Autodesk Fusion 360 part; units mm, degrees
note: some values were not read from the file. Set by a fixed rule: which sketch regions a step uses.
(part 27 of 59)
  spline S36 degree 5 poles (-3.9508, -16.2753) (-3.9508, -16.2754) (-3.9508, -16.2756) (-3.9509, -16.2759) (-3.9509, -16.2764) (-3.951, -16.2772) (-3.9511, -16.278) (-3.9512, -16.279) (-3.9514, -16.2801) (-3.9515, -16.2813) (-3.9517, -16.2826) (-3.9518, -16.284) (-3.952, -16.2855) (-3.9522, -16.2871) (-3.9523, -16.2889) (-3.9525, -16.2907) (-3.9527, -16.2926) (-3.9529, -16.2946) (-3.9531, -16.2968) (-3.9534, -16.299) (-3.9536, -16.3013) (-3.9538, -16.3037) (-3.954, -16.3063) (-3.9543, -16.3089) (-3.9545, -16.3116) (-3.9547, -16.3144) (-3.955, -16.3172) (-3.9552, -16.3202) (-3.9555, -16.3233) (-3.9557, -16.3264) (-3.9559, -16.3297) (-3.9562, -16.333) (-3.9564, -16.3364) (-3.9567, -16.3399) (-3.9569, -16.3435) (-3.9572, -16.3472) (-3.9574, -16.3509) (-3.9577, -16.3547) (-3.9579, -16.3586) (-3.9581, -16.3626) (-3.9584, -16.3667) (-3.9586, -16.3709) (-3.9588, -16.3751) (-3.959, -16.3794) (-3.9593, -16.3838) (-3.9595, -16.3882) (-3.9597, -16.3928) (-3.9599, -16.3974) (-3.9601, -16.4021) (-3.9603, -16.4068) (-3.9605, -16.4117) (-3.9607, -16.4166) (-3.9609, -16.4215) (-3.961, -16.4266) (-3.9612, -16.4317) (-3.9614, -16.4369) (-3.9615, -16.4422) (-3.9617, -16.4475) (-3.9618, -16.4529) (-3.962, -16.4584) (-3.9621, -16.4639) (-3.9622, -16.4695) (-3.9623, -16.4752) (-3.9624, -16.4809) (-3.9625, -16.4867) (-3.9626, -16.4926) (-3.9627, -16.4985) (-3.9627, -16.5045) (-3.9628, -16.5106) (-3.9629, -16.5167) (-3.9629, -16.5229) (-3.9629, -16.5291) (-3.9629, -16.5355) (-3.963, -16.5418) (-3.963, -16.5483) (-3.9629, -16.5548) (-3.9629, -16.5613) (-3.9629, -16.568) (-3.9628, -16.5746) (-3.9628, -16.5814) (-3.9627, -16.5882) (-3.9626, -16.595) (-3.9626, -16.6019) (-3.9625, -16.6089) (-3.9623, -16.6159) (-3.9622, -16.623) (-3.9621, -16.6302) (-3.9619, -16.6374) (-3.9618, -16.6446) (-3.9616, -16.6519) (-3.9614, -16.6593) (-3.9612, -16.6667) (-3.961, -16.6742) (-3.9607, -16.6817) (-3.9605, -16.6893) (-3.9603, -16.697) (-3.96, -16.7047) (-3.9597, -16.7124) (-3.9594, -16.7202) (-3.9591, -16.7281) (-3.9588, -16.736) (-3.9584, -16.7439) (-3.9581, -16.7519) (-3.9577, -16.76) (-3.9573, -16.7681) (-3.9569, -16.7763) (-3.9565, -16.7845) (-3.9561, -16.7927) (-3.9556, -16.801) (-3.9552, -16.8094) (-3.9547, -16.8178) (-3.9542, -16.8263) (-3.9537, -16.8348) (-3.9532, -16.8433) (-3.9526, -16.8519) (-3.9521, -16.8606) (-3.9515, -16.8693) (-3.9509, -16.878) (-3.9503, -16.8868) (-3.9497, -16.8957) (-3.9491, -16.9045) (-3.9484, -16.9135) (-3.9478, -16.9225) (-3.9471, -16.9315) (-3.9464, -16.9406) (-3.9457, -16.9497) (-3.9449, -16.9588) (-3.9442, -16.968) (-3.9434, -16.9773) (-3.9426, -16.9866) (-3.9418, -16.9959) (-3.941, -17.0053) (-3.9402, -17.0147) (-3.9393, -17.0242) (-3.9384, -17.0337) (-3.9375, -17.0433) (-3.9366, -17.0529) (-3.9357, -17.0625) (-3.9348, -17.0722) (-3.9338, -17.0819) (-3.9328, -17.0917) (-3.9318, -17.1015) (-3.9308, -17.1113) (-3.9297, -17.1212) (-3.9287, -17.1312) (-3.9276, -17.1411) (-3.9265, -17.1512) (-3.9254, -17.1612) (-3.9243, -17.1713) (-3.9231, -17.1814) (-3.922, -17.1916) (-3.9208, -17.2018) (-3.9196, -17.2121) (-3.9183, -17.2224) (-3.9171, -17.2327) (-3.9158, -17.2431) (-3.9145, -17.2535) (-3.9132, -17.264) (-3.9119, -17.2744) (-3.9106, -17.285) (-3.9092, -17.2955) (-3.9078, -17.3061) (-3.9064, -17.3168) (-3.905, -17.3274) (-3.9035, -17.3382) (-3.9021, -17.3489) (-3.9006, -17.3597) (-3.8991, -17.3705) (-3.8976, -17.3814) (-3.896, -17.3923) (-3.8945, -17.4032) (-3.8929, -17.4142) (-3.8913, -17.4252) (-3.8896, -17.4362) (-3.888, -17.4473) (-3.8863, -17.4584) (-3.8846, -17.4696) (-3.8829, -17.4807) (-3.8812, -17.492) (-3.8795, -17.5032) (-3.8777, -17.5145) (-3.8759, -17.5258) (-3.8741, -17.5372) (-3.8722, -17.5486) (-3.8704, -17.56) (-3.8685, -17.5714) (-3.8666, -17.5829) (-3.8647, -17.5944) (-3.8628, -17.606) (-3.8608, -17.6176) (-3.8588, -17.6292) (-3.8568, -17.6409) (-3.8548, -17.6525) (-3.8527, -17.6643) (-3.8507, -17.676) (-3.8486, -17.6878) (-3.8464, -17.6996) (-3.8443, -17.7115) (-3.8422, -17.7233) (-3.84, -17.7353) (-3.8378, -17.7472) (-3.8356, -17.7592) (-3.8333, -17.7712) (-3.831, -17.7832) (-3.8288, -17.7953) (-3.8264, -17.8074) (-3.8241, -17.8195) (-3.8217, -17.8317) (-3.8194, -17.8439) (-3.817, -17.8561) (-3.8145, -17.8683) (-3.8121, -17.8806) (-3.8096, -17.8929) (-3.8071, -17.9053) (-3.8046, -17.9176) (-3.8021, -17.93) (-3.7995, -17.9424) (-3.797, -17.9549) (-3.7943, -17.9674) (-3.7917, -17.9799) (-3.7891, -17.9924) (-3.7864, -18.005) (-3.7837, -18.0176) (-3.781, -18.0302) (-3.7782, -18.0429) (-3.7755, -18.0556) (-3.7727, -18.0683) (-3.7699, -18.081) (-3.767, -18.0938) (-3.7642, -18.1066) (-3.7613, -18.1194) (-3.7584, -18.1323) (-3.7555, -18.1451) (-3.7525, -18.158) (-3.7496, -18.171) (-3.7466, -18.1839) (-3.7435, -18.1969) (-3.7405, -18.2099) (-3.7374, -18.223) (-3.7343, -18.236) (-3.7312, -18.2491) (-3.7287, -18.2596) (-3.7268, -18.2675) (-3.7256, -18.2728) (-3.7249, -18.2754) knots 0 0 0 0 0 0 0.00416667 0.00833333 0.0125 0.01666667 0.02083333 0.025 0.02916667 0.03333333 0.0375 0.04166667 0.04583333 0.05 0.05416667 0.05833333 0.0625 0.06666667 0.07083333 0.075 0.07916667 0.08333333 0.0875 0.09166667 0.09583333 0.1 0.10416667 0.10833333 0.1125 0.11666667 0.12083333 0.125 0.12916667 0.13333333 0.1375 0.14166667 0.14583333 0.15 0.15416667 0.15833333 0.1625 0.16666667 0.17083333 0.175 0.17916667 0.18333333 0.1875 0.19166667 0.19583333 0.2 0.20416667 0.20833333 0.2125 0.21666667 0.22083333 0.225 0.22916667 0.23333333 0.2375 0.24166667 0.24583333 0.25 0.25416667 0.25833333 0.2625 0.26666667 0.27083333 0.275 0.27916667 0.28333333 0.2875 0.29166667 0.29583333 0.3 0.30416667 0.30833333 0.3125 0.31666667 0.32083333 0.325 0.32916667 0.33333333 0.3375 0.34166667 0.34583333 0.35 0.35416667 0.35833333 0.3625 0.36666667 0.37083333 0.375 0.37916667 0.38333333 0.3875 0.39166667 0.39583333 0.4 0.40416667 0.40833333 0.4125 0.41666667 0.42083333 0.425 0.42916667 0.43333333 0.4375 0.44166667 0.44583333 0.45 0.45416667 0.45833333 0.4625 0.46666667 0.47083333 0.475 0.47916667 0.48333333 0.4875 0.49166667 0.49583333 0.5 0.50416667 0.50833333 0.5125 0.51666667 0.52083333 0.525 0.52916667 0.53333333 0.5375 0.54166667 0.54583333 0.55 0.55416667 0.55833333 0.5625 0.56666667 0.57083333 0.575 0.57916667 0.58333333 0.5875 0.59166667 0.59583333 0.6 0.60416667 0.60833333 0.6125 0.61666667 0.62083333 0.625 0.62916667 0.63333333 0.6375 0.64166667 0.64583333 0.65 0.65416667 0.65833333 0.6625 0.66666667 0.67083333 0.675 0.67916667 0.68333333 0.6875 0.69166667 0.69583333 0.7 0.70416667 0.70833333 0.7125 0.71666667 0.72083333 0.725 0.72916667 0.73333333 0.7375 0.74166667 0.74583333 0.75 0.75416667 0.75833333 0.7625 0.76666667 0.77083333 0.775 0.77916667 0.78333333 0.7875 0.79166667 0.79583333 0.8 0.80416667 0.80833333 0.8125 0.81666667 0.82083333 0.825 0.82916667 0.83333333 0.8375 0.84166667 0.84583333 0.85 0.85416667 0.85833333 0.8625 0.86666667 0.87083333 0.875 0.87916667 0.88333333 0.8875 0.89166667 0.89583333 0.9 0.90416667 0.90833333 0.9125 0.91666667 0.92083333 0.925 0.92916667 0.93333333 0.9375 0.94166667 0.94583333 0.95 0.95416667 0.95833333 0.9625 0.96666667 0.97083333 0.975 0.97916667 0.98333333 0.9875 0.99166667 0.99583333 1 1 1 1 1 1
  arc A45 (-3.7249, -18.2754) -> (-2.755, -18.3773) centre (0, 12.5) ccw
  spline S37 degree 5 poles (-2.755, -18.3773) (-2.7539, -18.3749) (-2.7515, -18.37) (-2.748, -18.3627) (-2.7434, -18.353) (-2.7376, -18.3408) (-2.7319, -18.3287) (-2.7262, -18.3165) (-2.7205, -18.3044) (-2.7149, -18.2924) (-2.7092, -18.2803) (-2.7036, -18.2683) (-2.6981, -18.2563) (-2.6925, -18.2443) (-2.687, -18.2323) (-2.6815, -18.2204) (-2.6761, -18.2085) (-2.6707, -18.1966) (-2.6653, -18.1847) (-2.6599, -18.1728) (-2.6545, -18.161) (-2.6492, -18.1492) (-2.6439, -18.1374) (-2.6387, -18.1256) (-2.6335, -18.1139) (-2.6283, -18.1022) (-2.6231, -18.0905) (-2.6179, -18.0788) (-2.6128, -18.0672) (-2.6077, -18.0555) (-2.6027, -18.0439) (-2.5977, -18.0324) (-2.5927, -18.0208) (-2.5877, -18.0093) (-2.5827, -17.9978) (-2.5778, -17.9863) (-2.5729, -17.9749) (-2.5681, -17.9634) (-2.5632, -17.952) (-2.5584, -17.9407) (-2.5537, -17.9293) (-2.5489, -17.918) (-2.5442, -17.9067) (-2.5395, -17.8954) (-2.5348, -17.8841) (-2.5302, -17.8729) (-2.5256, -17.8617) (-2.521, -17.8506) (-2.5165, -17.8394) (-2.5119, -17.8283) (-2.5074, -17.8172) (-2.503, -17.8061) (-2.4985, -17.7951) (-2.4941, -17.7841) (-2.4897, -17.7731) (-2.4854, -17.7621) (-2.481, -17.7512) (-2.4767, -17.7403) (-2.4725, -17.7294) (-2.4682, -17.7186) (-2.464, -17.7078) (-2.4598, -17.697) (-2.4557, -17.6862) (-2.4515, -17.6755) (-2.4474, -17.6648) (-2.4433, -17.6541) (-2.4393, -17.6435) (-2.4353, -17.6329) (-2.4313, -17.6223) (-2.4273, -17.6118) (-2.4234, -17.6012) (-2.4194, -17.5907) (-2.4156, -17.5803) (-2.4117, -17.5699) (-2.4079, -17.5595) (-2.4041, -17.5491) (-2.4003, -17.5388) (-2.3965, -17.5284) (-2.3928, -17.5182) (-2.3891, -17.5079) (-2.3855, -17.4977) (-2.3818, -17.4875) (-2.3782, -17.4774) (-2.3746, -17.4673) (-2.3711, -17.4572) (-2.3675, -17.4471) (-2.364, -17.4371) (-2.3606, -17.4271) (-2.3571, -17.4172) (-2.3537, -17.4073) (-2.3503, -17.3974) (-2.3469, -17.3875) (-2.3436, -17.3777) (-2.3403, -17.368) (-2.337, -17.3582) (-2.3337, -17.3485) (-2.3305, -17.3388) (-2.3273, -17.3292) (-2.3241, -17.3196) (-2.321, -17.31) (-2.3178, -17.3005) (-2.3147, -17.291) (-2.3117, -17.2815) (-2.3086, -17.2721) (-2.3056, -17.2627) (-2.3026, -17.2534) (-2.2996, -17.2441) (-2.2967, -17.2348) (-2.2938, -17.2255) (-2.2909, -17.2163) (-2.288, -17.2072) (-2.2852, -17.1981) (-2.2824, -17.189) (-2.2796, -17.1799) (-2.2769, -17.1709) (-2.2741, -17.1619) (-2.2714, -17.153) (-2.2688, -17.1441) (-2.2661, -17.1353) (-2.2635, -17.1265) (-2.2609, -17.1177) (-2.2583, -17.109) (-2.2558, -17.1003) (-2.2533, -17.0917) (-2.2508, -17.083) (-2.2483, -17.0745) (-2.2458, -17.066) (-2.2434, -17.0575) (-2.241, -17.0491) (-2.2387, -17.0407) (-2.2363, -17.0323) (-2.234, -17.024) (-2.2317, -17.0158) (-2.2295, -17.0075) (-2.2272, -16.9994) (-2.225, -16.9912) (-2.2228, -16.9832) (-2.2207, -16.9751) (-2.2185, -16.9671) (-2.2164, -16.9592) (-2.2143, -16.9513) (-2.2123, -16.9434) (-2.2102, -16.9356) (-2.2082, -16.9279) (-2.2062, -16.9202) (-2.2043, -16.9125) (-2.2023, -16.9049) (-2.2004, -16.8973) (-2.1985, -16.8898) (-2.1967, -16.8823) (-2.1948, -16.8749) (-2.193, -16.8675) (-2.1912, -16.8602) (-2.1895, -16.8529) (-2.1877, -16.8457) (-2.186, -16.8386) (-2.1843, -16.8314) (-2.1827, -16.8244) (-2.181, -16.8174) (-2.1794, -16.8104) (-2.1778, -16.8035) (-2.1762, -16.7967) (-2.1747, -16.7899) (-2.1731, -16.7831) (-2.1716, -16.7764) (-2.1702, -16.7698) (-2.1687, -16.7632) (-2.1673, -16.7567) (-2.1659, -16.7502) (-2.1645, -16.7438) (-2.1631, -16.7374) (-2.1618, -16.7311) (-2.1605, -16.7249) (-2.1592, -16.7187) (-2.1579, -16.7126) (-2.1567, -16.7065) (-2.1554, -16.7005) (-2.1542, -16.6946) (-2.153, -16.6887) (-2.1519, -16.6829) (-2.1507, -16.6771) (-2.1496, -16.6714) (-2.1485, -16.6658) (-2.1475, -16.6602) (-2.1464, -16.6547) (-2.1454, -16.6493) (-2.1444, -16.6439) (-2.1434, -16.6386) (-2.1424, -16.6334) (-2.1415, -16.6282) (-2.1406, -16.6231) (-2.1397, -16.618) (-2.1388, -16.6131) (-2.138, -16.6081) (-2.1371, -16.6033) (-2.1363, -16.5985) (-2.1355, -16.5938) (-2.1347, -16.5892) (-2.134, -16.5847) (-2.1332, -16.5802) (-2.1325, -16.5758) (-2.1318, -16.5714) (-2.1312, -16.5672) (-2.1305, -16.563) (-2.1299, -16.5589) (-2.1292, -16.5549) (-2.1286, -16.5509) (-2.1281, -16.547) (-2.1275, -16.5432) (-2.127, -16.5395) (-2.1264, -16.5359) (-2.1259, -16.5323) (-2.1254, -16.5289) (-2.125, -16.5255) (-2.1245, -16.5222) (-2.1241, -16.5189) (-2.1237, -16.5158) (-2.1233, -16.5128) (-2.1229, -16.5098) (-2.1225, -16.5069) (-2.1222, -16.5041) (-2.1219, -16.5015) (-2.1215, -16.4989) (-2.1212, -16.4963) (-2.121, -16.4939) (-2.1207, -16.4916) (-2.1204, -16.4894) (-2.1202, -16.4873) (-2.12, -16.4852) (-2.1198, -16.4833) (-2.1196, -16.4815) (-2.1194, -16.4798) (-2.1192, -16.4781) (-2.1191, -16.4766) (-2.1189, -16.4752) (-2.1188, -16.4739) (-2.1187, -16.4727) (-2.1186, -16.4716) (-2.1185, -16.4706) (-2.1184, -16.4698) (-2.1184, -16.469) (-2.1183, -16.4685) (-2.1183, -16.4682) (-2.1183, -16.468) (-2.1183, -16.4679) knots -1 -1 -1 -1 -1 -1 -0.99583333 -0.99166667 -0.9875 -0.98333333 -0.97916667 -0.975 -0.97083333 -0.96666667 -0.9625 -0.95833333 -0.95416667 -0.95 -0.94583333 -0.94166667 -0.9375 -0.93333333 -0.92916667 -0.925 -0.92083333 -0.91666667 -0.9125 -0.90833333 -0.90416667 -0.9 -0.89583333 -0.89166667 -0.8875 -0.88333333 -0.87916667 -0.875 -0.87083333 -0.86666667 -0.8625 -0.85833333 -0.85416667 -0.85 -0.84583333 -0.84166667 -0.8375 -0.83333333 -0.82916667 -0.825 -0.82083333 -0.81666667 -0.8125 -0.80833333 -0.80416667 -0.8 -0.79583333 -0.79166667 -0.7875 -0.78333333 -0.77916667 -0.775 -0.77083333 -0.76666667 -0.7625 -0.75833333 -0.75416667 -0.75 -0.74583333 -0.74166667 -0.7375 -0.73333333 -0.72916667 -0.725 -0.72083333 -0.71666667 -0.7125 -0.70833333 -0.70416667 -0.7 -0.69583333 -0.69166667 -0.6875 -0.68333333 -0.67916667 -0.675 -0.67083333 -0.66666667 -0.6625 -0.65833333 -0.65416667 -0.65 -0.64583333 -0.64166667 -0.6375 -0.63333333 -0.62916667 -0.625 -0.62083333 -0.61666667 -0.6125 -0.60833333 -0.60416667 -0.6 -0.59583333 -0.59166667 -0.5875 -0.58333333 -0.57916667 -0.575 -0.57083333 -0.56666667 -0.5625 -0.55833333 -0.55416667 -0.55 -0.54583333 -0.54166667 -0.5375 -0.53333333 -0.52916667 -0.525 -0.52083333 -0.51666667 -0.5125 -0.50833333 -0.50416667 -0.5 -0.49583333 -0.49166667 -0.4875 -0.48333333 -0.47916667 -0.475 -0.47083333 -0.46666667 -0.4625 -0.45833333 -0.45416667 -0.45 -0.44583333 -0.44166667 -0.4375 -0.43333333 -0.42916667 -0.425 -0.42083333 -0.41666667 -0.4125 -0.40833333 -0.40416667 -0.4 -0.39583333 -0.39166667 -0.3875 -0.38333333 -0.37916667 -0.375 -0.37083333 -0.36666667 -0.3625 -0.35833333 -0.35416667 -0.35 -0.34583333 -0.34166667 -0.3375 -0.33333333 -0.32916667 -0.325 -0.32083333 -0.31666667 -0.3125 -0.30833333 -0.30416667 -0.3 -0.29583333 -0.29166667 -0.2875 -0.28333333 -0.27916667 -0.275 -0.27083333 -0.26666667 -0.2625 -0.25833333 -0.25416667 -0.25 -0.24583333 -0.24166667 -0.2375 -0.23333333 -0.22916667 -0.225 -0.22083333 -0.21666667 -0.2125 -0.20833333 -0.20416667 -0.2 -0.19583333 -0.19166667 -0.1875 -0.18333333 -0.17916667 -0.175 -0.17083333 -0.16666667 -0.1625 -0.15833333 -0.15416667 -0.15 -0.14583333 -0.14166667 -0.1375 -0.13333333 -0.12916667 -0.125 -0.12083333 -0.11666667 -0.1125 -0.10833333 -0.10416667 -0.1 -0.09583333 -0.09166667 -0.0875 -0.08333333 -0.07916667 -0.075 -0.07083333 -0.06666667 -0.0625 -0.05833333 -0.05416667 -0.05 -0.04583333 -0.04166667 -0.0375 -0.03333333 -0.02916667 -0.025 -0.02083333 -0.01666667 -0.0125 -0.00833333 -0.00416667 0 0 0 0 0 0
  line L75 (-2.1183, -16.4679) -> (-2.1182, -16.4671)
  line L76 (-2.1182, -16.4671) -> (-2.0967, -16.1734)
  arc A46 (-2.0967, -16.1734) -> (-0.9119, -16.2355) centre (0, 12.5) ccw
  line L77 (-0.9119, -16.2355) -> (-0.9213, -16.5298)
  line L78 (-0.9213, -16.5298) -> (-0.9213, -16.5307)
  spline S38 degree 5 poles (-0.9213, -16.5307) (-0.9213, -16.5307) (-0.9213, -16.5309) (-0.9213, -16.5313) (-0.9213, -16.5318) (-0.9213, -16.5325) (-0.9213, -16.5334) (-0.9214, -16.5344) (-0.9214, -16.5355) (-0.9214, -16.5367) (-0.9214, -16.538) (-0.9214, -16.5394) (-0.9214, -16.5409) (-0.9214, -16.5425) (-0.9214, -16.5443) (-0.9214, -16.5461) (-0.9214, -16.5481) (-0.9214, -16.5501) (-0.9214, -16.5522) (-0.9214, -16.5545) (-0.9214, -16.5568) (-0.9213, -16.5592) (-0.9213, -16.5618) (-0.9212, -16.5644) (-0.9212, -16.5671) (-0.9211, -16.5699) (-0.9211, -16.5728) (-0.921, -16.5758) (-0.9209, -16.5788) (-0.9208, -16.582) (-0.9208, -16.5852) (-0.9206, -16.5886) (-0.9205, -16.592) (-0.9204, -16.5955) (-0.9203, -16.5991) (-0.9201, -16.6028) (-0.92, -16.6065) (-0.9198, -16.6103) (-0.9197, -16.6143) (-0.9195, -16.6183) (-0.9193, -16.6223) (-0.9191, -16.6265) (-0.9189, -16.6307) (-0.9186, -16.635) (-0.9184, -16.6394) (-0.9182, -16.6439) (-0.9179, -16.6484) (-0.9176, -16.653) (-0.9173, -16.6577) (-0.917, -16.6624) (-0.9167, -16.6673) (-0.9164, -16.6722) (-0.9161, -16.6771) (-0.9157, -16.6822) (-0.9153, -16.6873) (-0.915, -16.6925) (-0.9146, -16.6977) (-0.9141, -16.703) (-0.9137, -16.7084) (-0.9133, -16.7139) (-0.9128, -16.7194) (-0.9124, -16.725) (-0.9119, -16.7306) (-0.9114, -16.7363) (-0.9109, -16.7421) (-0.9103, -16.748) (-0.9098, -16.7539) (-0.9092, -16.7599) (-0.9087, -16.7659) (-0.9081, -16.772) (-0.9075, -16.7781) (-0.9068, -16.7844) (-0.9062, -16.7906) (-0.9055, -16.797) (-0.9049, -16.8034) (-0.9042, -16.8099) (-0.9035, -16.8164) (-0.9027, -16.823) (-0.902, -16.8296) (-0.9012, -16.8363) (-0.9005, -16.843) (-0.8997, -16.8498) (-0.8989, -16.8567) (-0.898, -16.8636) (-0.8972, -16.8706) (-0.8963, -16.8777) (-0.8954, -16.8847) (-0.8945, -16.8919) (-0.8936, -16.8991) (-0.8927, -16.9063) (-0.8917, -16.9137) (-0.8907, -16.921) (-0.8897, -16.9284) (-0.8887, -16.9359) (-0.8877, -16.9434) (-0.8866, -16.951) (-0.8856, -16.9586) (-0.8845, -16.9663) (-0.8834, -16.974) (-0.8822, -16.9818) (-0.8811, -16.9896) (-0.8799, -16.9975) (-0.8787, -17.0054) (-0.8775, -17.0134) (-0.8763, -17.0214) (-0.875, -17.0295) (-0.8738, -17.0376) (-0.8725, -17.0458) (-0.8712, -17.054) (-0.8698, -17.0623) (-0.8685, -17.0706) (-0.8671, -17.0789) (-0.8657, -17.0873) (-0.8643, -17.0958) (-0.8629, -17.1043) (-0.8614, -17.1128) (-0.86, -17.1214) (-0.8585, -17.1301) (-0.8569, -17.1388) (-0.8554, -17.1475) (-0.8538, -17.1563) (-0.8523, -17.1651) (-0.8507, -17.1739) (-0.849, -17.1828) (-0.8474, -17.1918) (-0.8457, -17.2008) (-0.844, -17.2098) (-0.8423, -17.2189) (-0.8406, -17.228) (-0.8388, -17.2372) (-0.8371, -17.2464) (-0.8353, -17.2556) (-0.8334, -17.2649) (-0.8316, -17.2742) (-0.8297, -17.2836) (-0.8279, -17.293) (-0.8259, -17.3025) (-0.824, -17.312) (-0.8221, -17.3215) (-0.8201, -17.3311) (-0.8181, -17.3407) (-0.8161, -17.3503) (-0.814, -17.36) (-0.812, -17.3697) (-0.8099, -17.3795) (-0.8078, -17.3893) (-0.8056, -17.3992) (-0.8035, -17.409) (-0.8013, -17.419) (-0.7991, -17.4289) (-0.7969, -17.4389) (-0.7946, -17.449) (-0.7923, -17.459) (-0.79, -17.4691) (-0.7877, -17.4793) (-0.7854, -17.4895) (-0.783, -17.4997) (-0.7806, -17.5099) (-0.7782, -17.5202) (-0.7758, -17.5306) (-0.7733, -17.5409) (-0.7708, -17.5513) (-0.7683, -17.5618) (-0.7658, -17.5722) (-0.7632, -17.5827) (-0.7606, -17.5933) (-0.758, -17.6038) (-0.7554, -17.6145) (-0.7528, -17.6251) (-0.7501, -17.6358) (-0.7474, -17.6465) (-0.7447, -17.6572) (-0.7419, -17.668) (-0.7391, -17.6788) (-0.7364, -17.6897) (-0.7335, -17.7005) (-0.7307, -17.7114) (-0.7278, -17.7224) (-0.7249, -17.7334) (-0.722, -17.7444) (-0.7191, -17.7554) (-0.7161, -17.7665) (-0.7131, -17.7776) (-0.7101, -17.7887) (-0.7071, -17.7999) (-0.704, -17.8111) (-0.7009, -17.8223) (-0.6978, -17.8336) (-0.6947, -17.8448) (-0.6915, -17.8562) (-0.6883, -17.8675) (-0.6851, -17.8789) (-0.6819, -17.8903) (-0.6786, -17.9017) (-0.6753, -17.9132) (-0.672, -17.9247) (-0.6687, -17.9362) (-0.6653, -17.9478) (-0.6619, -17.9594) (-0.6585, -17.971) (-0.6551, -17.9827) (-0.6516, -17.9943) (-0.6481, -18.006) (-0.6446, -18.0178) (-0.6411, -18.0295) (-0.6375, -18.0413) (-0.6339, -18.0531) (-0.6303, -18.065) (-0.6267, -18.0769) (-0.623, -18.0888) (-0.6193, -18.1007) (-0.6156, -18.1126) (-0.6118, -18.1246) (-0.6081, -18.1366) (-0.6043, -18.1487) (-0.6005, -18.1607) (-0.5966, -18.1728) (-0.5927, -18.185) (-0.5889, -18.1971) (-0.5849, -18.2093) (-0.581, -18.2215) (-0.577, -18.2337) (-0.573, -18.2459) (-0.569, -18.2582) (-0.5649, -18.2705) (-0.5609, -18.2828) (-0.5568, -18.2952) (-0.5526, -18.3076) (-0.5485, -18.32) (-0.5443, -18.3324) (-0.5401, -18.3448) (-0.5359, -18.3573) (-0.5316, -18.3698) (-0.5273, -18.3823) (-0.523, -18.3949) (-0.5187, -18.4075) (-0.5143, -18.4201) (-0.5099, -18.4327) (-0.5055, -18.4453) (-0.5011, -18.458) (-0.4966, -18.4707) (-0.493, -18.4809) (-0.4903, -18.4885) (-0.4885, -18.4936) (-0.4876, -18.4962) knots 0 0 0 0 0 0 0.00416667 0.00833333 0.0125 0.01666667 0.02083333 0.025 0.02916667 0.03333333 0.0375 0.04166667 0.04583333 0.05 0.05416667 0.05833333 0.0625 0.06666667 0.07083333 0.075 0.07916667 0.08333333 0.0875 0.09166667 0.09583333 0.1 0.10416667 0.10833333 0.1125 0.11666667 0.12083333 0.125 0.12916667 0.13333333 0.1375 0.14166667 0.14583333 0.15 0.15416667 0.15833333 0.1625 0.16666667 0.17083333 0.175 0.17916667 0.18333333 0.1875 0.19166667 0.19583333 0.2 0.20416667 0.20833333 0.2125 0.21666667 0.22083333 0.225 0.22916667 0.23333333 0.2375 0.24166667 0.24583333 0.25 0.25416667 0.25833333 0.2625 0.26666667 0.27083333 0.275 0.27916667 0.28333333 0.2875 0.29166667 0.29583333 0.3 0.30416667 0.30833333 0.3125 0.31666667 0.32083333 0.325 0.32916667 0.33333333 0.3375 0.34166667 0.34583333 0.35 0.35416667 0.35833333 0.3625 0.36666667 0.37083333 0.375 0.37916667 0.38333333 0.3875 0.39166667 0.39583333 0.4 0.40416667 0.40833333 0.4125 0.41666667 0.42083333 0.425 0.42916667 0.43333333 0.4375 0.44166667 0.44583333 0.45 0.45416667 0.45833333 0.4625 0.46666667 0.47083333 0.475 0.47916667 0.48333333 0.4875 0.49166667 0.49583333 0.5 0.50416667 0.50833333 0.5125 0.51666667 0.52083333 0.525 0.52916667 0.53333333 0.5375 0.54166667 0.54583333 0.55 0.55416667 0.55833333 0.5625 0.56666667 0.57083333 0.575 0.57916667 0.58333333 0.5875 0.59166667 0.59583333 0.6 0.60416667 0.60833333 0.6125 0.61666667 0.62083333 0.625 0.62916667 0.63333333 0.6375 0.64166667 0.64583333 0.65 0.65416667 0.65833333 0.6625 0.66666667 0.67083333 0.675 0.67916667 0.68333333 0.6875 0.69166667 0.69583333 0.7 0.70416667 0.70833333 0.7125 0.71666667 0.72083333 0.725 0.72916667 0.73333333 0.7375 0.74166667 0.74583333 0.75 0.75416667 0.75833333 0.7625 0.76666667 0.77083333 0.775 0.77916667 0.78333333 0.7875 0.79166667 0.79583333 0.8 0.80416667 0.80833333 0.8125 0.81666667 0.82083333 0.825 0.82916667 0.83333333 0.8375 0.84166667 0.84583333 0.85 0.85416667 0.85833333 0.8625 0.86666667 0.87083333 0.875 0.87916667 0.88333333 0.8875 0.89166667 0.89583333 0.9 0.90416667 0.90833333 0.9125 0.91666667 0.92083333 0.925 0.92916667 0.93333333 0.9375 0.94166667 0.94583333 0.95 0.95416667 0.95833333 0.9625 0.96666667 0.97083333 0.975 0.97916667 0.98333333 0.9875 0.99166667 0.99583333 1 1 1 1 1 1
  arc A47 (-0.4876, -18.4962) -> (0.4876, -18.4962) centre (0, 12.5) ccw
  spline S39 degree 5 poles (0.4876, -18.4962) (0.4885, -18.4936) (0.4903, -18.4885) (0.493, -18.4809) (0.4966, -18.4707) (0.5011, -18.458) (0.5055, -18.4453) (0.5099, -18.4327) (0.5143, -18.4201) (0.5187, -18.4075) (0.523, -18.3949) (0.5273, -18.3823) (0.5316, -18.3698) (0.5359, -18.3573) (0.5401, -18.3448) (0.5443, -18.3324) (0.5485, -18.32) (0.5526, -18.3076) (0.5568, -18.2952) (0.5609, -18.2828) (0.5649, -18.2705) (0.569, -18.2582) (0.573, -18.2459) (0.577, -18.2337) (0.581, -18.2215) (0.5849, -18.2093) (0.5889, -18.1971) (0.5927, -18.185) (0.5966, -18.1728) (0.6005, -18.1607) (0.6043, -18.1487) (0.6081, -18.1366) (0.6118, -18.1246) (0.6156, -18.1126) (0.6193, -18.1007) (0.623, -18.0888) (0.6267, -18.0769) (0.6303, -18.065) (0.6339, -18.0531) (0.6375, -18.0413) (0.6411, -18.0295) (0.6446, -18.0178) (0.6481, -18.006) (0.6516, -17.9943) (0.6551, -17.9827) (0.6585, -17.971) (0.6619, -17.9594) (0.6653, -17.9478) (0.6687, -17.9362) (0.672, -17.9247) (0.6753, -17.9132) (0.6786, -17.9017) (0.6819, -17.8903) (0.6851, -17.8789) (0.6883, -17.8675) (0.6915, -17.8562) (0.6947, -17.8448) (0.6978, -17.8336) (0.7009, -17.8223) (0.704, -17.8111) (0.7071, -17.7999) (0.7101, -17.7887) (0.7131, -17.7776) (0.7161, -17.7665) (0.7191, -17.7554) (0.722, -17.7444) (0.7249, -17.7334) (0.7278, -17.7224) (0.7307, -17.7114) (0.7335, -17.7005) (0.7364, -17.6897) (0.7391, -17.6788) (0.7419, -17.668) (0.7447, -17.6572) (0.7474, -17.6465) (0.7501, -17.6358) (0.7528, -17.6251) (0.7554, -17.6145) (0.758, -17.6038) (0.7606, -17.5933) (0.7632, -17.5827) (0.7658, -17.5722) (0.7683, -17.5618) (0.7708, -17.5513) (0.7733, -17.5409) (0.7758, -17.5306) (0.7782, -17.5202) (0.7806, -17.5099) (0.783, -17.4997) (0.7854, -17.4895) (0.7877, -17.4793) (0.79, -17.4691) (0.7923, -17.459) (0.7946, -17.449) (0.7969, -17.4389) (0.7991, -17.4289) (0.8013, -17.419) (0.8035, -17.409) (0.8056, -17.3992) (0.8078, -17.3893) (0.8099, -17.3795) (0.812, -17.3697) (0.814, -17.36) (0.8161, -17.3503) (0.8181, -17.3407) (0.8201, -17.3311) (0.8221, -17.3215) (0.824, -17.312) (0.8259, -17.3025) (0.8279, -17.293) (0.8297, -17.2836) (0.8316, -17.2742) (0.8334, -17.2649) (0.8353, -17.2556) (0.8371, -17.2464) (0.8388, -17.2372) (0.8406, -17.228) (0.8423, -17.2189) (0.844, -17.2098) (0.8457, -17.2008) (0.8474, -17.1918) (0.849, -17.1828) (0.8507, -17.1739) (0.8523, -17.1651) (0.8538, -17.1563) (0.8554, -17.1475) (0.8569, -17.1388) (0.8585, -17.1301) (0.86, -17.1214) (0.8614, -17.1128) (0.8629, -17.1043) (0.8643, -17.0958) (0.8657, -17.0873) (0.8671, -17.0789) (0.8685, -17.0706) (0.8698, -17.0623) (0.8712, -17.054) (0.8725, -17.0458) (0.8738, -17.0376) (0.875, -17.0295) (0.8763, -17.0214) (0.8775, -17.0134) (0.8787, -17.0054) (0.8799, -16.9975) (0.8811, -16.9896) (0.8822, -16.9818) (0.8834, -16.974) (0.8845, -16.9663) (0.8856, -16.9586) (0.8866, -16.951) (0.8877, -16.9434) (0.8887, -16.9359) (0.8897, -16.9284) (0.8907, -16.921) (0.8917, -16.9137) (0.8927, -16.9063) (0.8936, -16.8991) (0.8945, -16.8919) (0.8954, -16.8847) (0.8963, -16.8777) (0.8972, -16.8706) (0.898, -16.8636) (0.8989, -16.8567) (0.8997, -16.8498) (0.9005, -16.843) (0.9012, -16.8363) (0.902, -16.8296) (0.9027, -16.823) (0.9035, -16.8164) (0.9042, -16.8099) (0.9049, -16.8034) (0.9055, -16.797) (0.9062, -16.7906) (0.9068, -16.7844) (0.9075, -16.7781) (0.9081, -16.772) (0.9087, -16.7659) (0.9092, -16.7599) (0.9098, -16.7539) (0.9103, -16.748) (0.9109, -16.7421) (0.9114, -16.7363) (0.9119, -16.7306) (0.9124, -16.725) (0.9128, -16.7194) (0.9133, -16.7139) (0.9137, -16.7084) (0.9141, -16.703) (0.9146, -16.6977) (0.915, -16.6925) (0.9153, -16.6873) (0.9157, -16.6822) (0.9161, -16.6771) (0.9164, -16.6722) (0.9167, -16.6673) (0.917, -16.6624) (0.9173, -16.6577) (0.9176, -16.653) (0.9179, -16.6484) (0.9182, -16.6439) (0.9184, -16.6394) (0.9186, -16.635) (0.9189, -16.6307) (0.9191, -16.6265) (0.9193, -16.6223) (0.9195, -16.6183) (0.9197, -16.6143) (0.9198, -16.6103) (0.92, -16.6065) (0.9201, -16.6028) (0.9203, -16.5991) (0.9204, -16.5955) (0.9205, -16.592) (0.9206, -16.5886) (0.9208, -16.5852) (0.9208, -16.582) (0.9209, -16.5788) (0.921, -16.5758) (0.9211, -16.5728) (0.9211, -16.5699) (0.9212, -16.5671) (0.9212, -16.5644) (0.9213, -16.5618) (0.9213, -16.5592) (0.9214, -16.5568) (0.9214, -16.5545) (0.9214, -16.5522) (0.9214, -16.5501) (0.9214, -16.5481) (0.9214, -16.5461) (0.9214, -16.5443) (0.9214, -16.5425) (0.9214, -16.5409) (0.9214, -16.5394) (0.9214, -16.538) (0.9214, -16.5367) (0.9214, -16.5355) (0.9214, -16.5344) (0.9213, -16.5334) (0.9213, -16.5325) (0.9213, -16.5318) (0.9213, -16.5313) (0.9213, -16.5309) (0.9213, -16.5307) (0.9213, -16.5307) knots -1 -1 -1 -1 -1 -1 -0.99583333 -0.99166667 -0.9875 -0.98333333 -0.97916667 -0.975 -0.97083333 -0.96666667 -0.9625 -0.95833333 -0.95416667 -0.95 -0.94583333 -0.94166667 -0.9375 -0.93333333 -0.92916667 -0.925 -0.92083333 -0.91666667 -0.9125 -0.90833333 -0.90416667 -0.9 -0.89583333 -0.89166667 -0.8875 -0.88333333 -0.87916667 -0.875 -0.87083333 -0.86666667 -0.8625 -0.85833333 -0.85416667 -0.85 -0.84583333 -0.84166667 -0.8375 -0.83333333 -0.82916667 -0.825 -0.82083333 -0.81666667 -0.8125 -0.80833333 -0.80416667 -0.8 -0.79583333 -0.79166667 -0.7875 -0.78333333 -0.77916667 -0.775 -0.77083333 -0.76666667 -0.7625 -0.75833333 -0.75416667 -0.75 -0.74583333 -0.74166667 -0.7375 -0.73333333 -0.72916667 -0.725 -0.72083333 -0.71666667 -0.7125 -0.70833333 -0.70416667 -0.7 -0.69583333 -0.69166667 -0.6875 -0.68333333 -0.67916667 -0.675 -0.67083333 -0.66666667 -0.6625 -0.65833333 -0.65416667 -0.65 -0.64583333 -0.64166667 -0.6375 -0.63333333 -0.62916667 -0.625 -0.62083333 -0.61666667 -0.6125 -0.60833333 -0.60416667 -0.6 -0.59583333 -0.59166667 -0.5875 -0.58333333 -0.57916667 -0.575 -0.57083333 -0.56666667 -0.5625 -0.55833333 -0.55416667 -0.55 -0.54583333 -0.54166667 -0.5375 -0.53333333 -0.52916667 -0.525 -0.52083333 -0.51666667 -0.5125 -0.50833333 -0.50416667 -0.5 -0.49583333 -0.49166667 -0.4875 -0.48333333 -0.47916667 -0.475 -0.47083333 -0.46666667 -0.4625 -0.45833333 -0.45416667 -0.45 -0.44583333 -0.44166667 -0.4375 -0.43333333 -0.42916667 -0.425 -0.42083333 -0.41666667 -0.4125 -0.40833333 -0.40416667 -0.4 -0.39583333 -0.39166667 -0.3875 -0.38333333 -0.37916667 -0.375 -0.37083333 -0.36666667 -0.3625 -0.35833333 -0.35416667 -0.35 -0.34583333 -0.34166667 -0.3375 -0.33333333 -0.32916667 -0.325 -0.32083333 -0.31666667 -0.3125 -0.30833333 -0.30416667 -0.3 -0.29583333 -0.29166667 -0.2875 -0.28333333 -0.27916667 -0.275 -0.27083333 -0.26666667 -0.2625 -0.25833333 -0.25416667 -0.25 -0.24583333 -0.24166667 -0.2375 -0.23333333 -0.22916667 -0.225 -0.22083333 -0.21666667 -0.2125 -0.20833333 -0.20416667 -0.2 -0.19583333 -0.19166667 -0.1875 -0.18333333 -0.17916667 -0.175 -0.17083333 -0.16666667 -0.1625 -0.15833333 -0.15416667 -0.15 -0.14583333 -0.14166667 -0.1375 -0.13333333 -0.12916667 -0.125 -0.12083333 -0.11666667 -0.1125 -0.10833333 -0.10416667 -0.1 -0.09583333 -0.09166667 -0.0875 -0.08333333 -0.07916667 -0.075 -0.07083333 -0.06666667 -0.0625 -0.05833333 -0.05416667 -0.05 -0.04583333 -0.04166667 -0.0375 -0.03333333 -0.02916667 -0.025 -0.02083333 -0.01666667 -0.0125 -0.00833333 -0.00416667 0 0 0 0 0 0
  line L79 (0.9213, -16.5307) -> (0.9213, -16.5298)
  line L80 (0.9213, -16.5298) -> (0.9119, -16.2355)
  arc A48 (0.9119, -16.2355) -> (2.0967, -16.1734) centre (0, 12.5) ccw
  line L81 (2.0967, -16.1734) -> (2.1182, -16.4671)
  line L82 (2.1182, -16.4671) -> (2.1183, -16.4679)
  spline S40 degree 5 poles (2.1183, -16.4679) (2.1183, -16.468) (2.1183, -16.4682) (2.1183, -16.4685) (2.1184, -16.469) (2.1184, -16.4698) (2.1185, -16.4706) (2.1186, -16.4716) (2.1187, -16.4727) (2.1188, -16.4739) (2.1189, -16.4752) (2.1191, -16.4766) (2.1192, -16.4781) (2.1194, -16.4798) (2.1196, -16.4815) (2.1198, -16.4833) (2.12, -16.4852) (2.1202, -16.4873) (2.1204, -16.4894) (2.1207, -16.4916) (2.121, -16.4939) (2.1212, -16.4963) (2.1215, -16.4989) (2.1219, -16.5015) (2.1222, -16.5041) (2.1225, -16.5069) (2.1229, -16.5098) (2.1233, -16.5128) (2.1237, -16.5158) (2.1241, -16.5189) (2.1245, -16.5222) (2.125, -16.5255) (2.1254, -16.5289) (2.1259, -16.5323) (2.1264, -16.5359) (2.127, -16.5395) (2.1275, -16.5432) (2.1281, -16.547) (2.1286, -16.5509) (2.1292, -16.5549) (2.1299, -16.5589) (2.1305, -16.563) (2.1312, -16.5672) (2.1318, -16.5714) (2.1325, -16.5758) (2.1332, -16.5802) (2.134, -16.5847) (2.1347, -16.5892) (2.1355, -16.5938) (2.1363, -16.5985) (2.1371, -16.6033) (2.138, -16.6081) (2.1388, -16.6131) (2.1397, -16.618) (2.1406, -16.6231) (2.1415, -16.6282) (2.1424, -16.6334) (2.1434, -16.6386) (2.1444, -16.6439) (2.1454, -16.6493) (2.1464, -16.6547) (2.1475, -16.6602) (2.1485, -16.6658) (2.1496, -16.6714) (2.1507, -16.6771) (2.1519, -16.6829) (2.153, -16.6887) (2.1542, -16.6946) (2.1554, -16.7005) (2.1567, -16.7065) (2.1579, -16.7126) (2.1592, -16.7187) (2.1605, -16.7249) (2.1618, -16.7311) (2.1631, -16.7374) (2.1645, -16.7438) (2.1659, -16.7502) (2.1673, -16.7567) (2.1687, -16.7632) (2.1702, -16.7698) (2.1716, -16.7764) (2.1731, -16.7831) (2.1747, -16.7899) (2.1762, -16.7967) (2.1778, -16.8035) (2.1794, -16.8104) (2.181, -16.8174) (2.1827, -16.8244) (2.1843, -16.8314) (2.186, -16.8386) (2.1877, -16.8457) (2.1895, -16.8529) (2.1912, -16.8602) (2.193, -16.8675) (2.1948, -16.8749) (2.1967, -16.8823) (2.1985, -16.8898) (2.2004, -16.8973) (2.2023, -16.9049) (2.2043, -16.9125) (2.2062, -16.9202) (2.2082, -16.9279) (2.2102, -16.9356) (2.2123, -16.9434) (2.2143, -16.9513) (2.2164, -16.9592) (2.2185, -16.9671) (2.2207, -16.9751) (2.2228, -16.9832) (2.225, -16.9912) (2.2272, -16.9994) (2.2295, -17.0075) (2.2317, -17.0158) (2.234, -17.024) (2.2363, -17.0323) (2.2387, -17.0407) (2.241, -17.0491) (2.2434, -17.0575) (2.2458, -17.066) (2.2483, -17.0745) (2.2508, -17.083) (2.2533, -17.0917) (2.2558, -17.1003) (2.2583, -17.109) (2.2609, -17.1177) (2.2635, -17.1265) (2.2661, -17.1353) (2.2688, -17.1441) (2.2714, -17.153) (2.2741, -17.1619) (2.2769, -17.1709) (2.2796, -17.1799) (2.2824, -17.189) (2.2852, -17.1981) (2.288, -17.2072) (2.2909, -17.2163) (2.2938, -17.2255) (2.2967, -17.2348) (2.2996, -17.2441) (2.3026, -17.2534) (2.3056, -17.2627) (2.3086, -17.2721) (2.3117, -17.2815) (2.3147, -17.291) (2.3178, -17.3005) (2.321, -17.31) (2.3241, -17.3196) (2.3273, -17.3292) (2.3305, -17.3388) (2.3337, -17.3485) (2.337, -17.3582) (2.3403, -17.368) (2.3436, -17.3777) (2.3469, -17.3875) (2.3503, -17.3974) (2.3537, -17.4073) (2.3571, -17.4172) (2.3606, -17.4271) (2.364, -17.4371) (2.3675, -17.4471) (2.3711, -17.4572) (2.3746, -17.4673) (2.3782, -17.4774) (2.3818, -17.4875) (2.3855, -17.4977) (2.3891, -17.5079) (2.3928, -17.5182) (2.3965, -17.5284) (2.4003, -17.5388) (2.4041, -17.5491) (2.4079, -17.5595) (2.4117, -17.5699) (2.4156, -17.5803) (2.4194, -17.5907) (2.4234, -17.6012) (2.4273, -17.6118) (2.4313, -17.6223) (2.4353, -17.6329) (2.4393, -17.6435) (2.4433, -17.6541) (2.4474, -17.6648) (2.4515, -17.6755) (2.4557, -17.6862) (2.4598, -17.697) (2.464, -17.7078) (2.4682, -17.7186) (2.4725, -17.7294) (2.4767, -17.7403) (2.481, -17.7512) (2.4854, -17.7621) (2.4897, -17.7731) (2.4941, -17.7841) (2.4985, -17.7951) (2.503, -17.8061) (2.5074, -17.8172) (2.5119, -17.8283) (2.5165, -17.8394) (2.521, -17.8506) (2.5256, -17.8617) (2.5302, -17.8729) (2.5348, -17.8841) (2.5395, -17.8954) (2.5442, -17.9067) (2.5489, -17.918) (2.5537, -17.9293) (2.5584, -17.9407) (2.5632, -17.952) (2.5681, -17.9634) (2.5729, -17.9749) (2.5778, -17.9863) (2.5827, -17.9978) (2.5877, -18.0093) (2.5927, -18.0208) (2.5977, -18.0324) (2.6027, -18.0439) (2.6077, -18.0555) (2.6128, -18.0672) (2.6179, -18.0788) (2.6231, -18.0905) (2.6283, -18.1022) (2.6335, -18.1139) (2.6387, -18.1256) (2.6439, -18.1374) (2.6492, -18.1492) (2.6545, -18.161) (2.6599, -18.1728) (2.6653, -18.1847) (2.6707, -18.1966) (2.6761, -18.2085) (2.6815, -18.2204) (2.687, -18.2323) (2.6925, -18.2443) (2.6981, -18.2563) (2.7036, -18.2683) (2.7092, -18.2803) (2.7149, -18.2924) (2.7205, -18.3044) (2.7262, -18.3165) (2.7319, -18.3287) (2.7376, -18.3408) (2.7434, -18.353) (2.748, -18.3627) (2.7515, -18.37) (2.7539, -18.3749) (2.755, -18.3773) knots 0 0 0 0 0 0 0.00416667 0.00833333 0.0125 0.01666667 0.02083333 0.025 0.02916667 0.03333333 0.0375 0.04166667 0.04583333 0.05 0.05416667 0.05833333 0.0625 0.06666667 0.07083333 0.075 0.07916667 0.08333333 0.0875 0.09166667 0.09583333 0.1 0.10416667 0.10833333 0.1125 0.11666667 0.12083333 0.125 0.12916667 0.13333333 0.1375 0.14166667 0.14583333 0.15 0.15416667 0.15833333 0.1625 0.16666667 0.17083333 0.175 0.17916667 0.18333333 0.1875 0.19166667 0.19583333 0.2 0.20416667 0.20833333 0.2125 0.21666667 0.22083333 0.225 0.22916667 0.23333333 0.2375 0.24166667 0.24583333 0.25 0.25416667 0.25833333 0.2625 0.26666667 0.27083333 0.275 0.27916667 0.28333333 0.2875 0.29166667 0.29583333 0.3 0.30416667 0.30833333 0.3125 0.31666667 0.32083333 0.325 0.32916667 0.33333333 0.3375 0.34166667 0.34583333 0.35 0.35416667 0.35833333 0.3625 0.36666667 0.37083333 0.375 0.37916667 0.38333333 0.3875 0.39166667 0.39583333 0.4 0.40416667 0.40833333 0.4125 0.41666667 0.42083333 0.425 0.42916667 0.43333333 0.4375 0.44166667 0.44583333 0.45 0.45416667 0.45833333 0.4625 0.46666667 0.47083333 0.475 0.47916667 0.48333333 0.4875 0.49166667 0.49583333 0.5 0.50416667 0.50833333 0.5125 0.51666667 0.52083333 0.525 0.52916667 0.53333333 0.5375 0.54166667 0.54583333 0.55 0.55416667 0.55833333 0.5625 0.56666667 0.57083333 0.575 0.57916667 0.58333333 0.5875 0.59166667 0.59583333 0.6 0.60416667 0.60833333 0.6125 0.61666667 0.62083333 0.625 0.62916667 0.63333333 0.6375 0.64166667 0.64583333 0.65 0.65416667 0.65833333 0.6625 0.66666667 0.67083333 0.675 0.67916667 0.68333333 0.6875 0.69166667 0.69583333 0.7 0.70416667 0.70833333 0.7125 0.71666667 0.72083333 0.725 0.72916667 0.73333333 0.7375 0.74166667 0.74583333 0.75 0.75416667 0.75833333 0.7625 0.76666667 0.77083333 0.775 0.77916667 0.78333333 0.7875 0.79166667 0.79583333 0.8 0.80416667 0.80833333 0.8125 0.81666667 0.82083333 0.825 0.82916667 0.83333333 0.8375 0.84166667 0.84583333 0.85 0.85416667 0.85833333 0.8625 0.86666667 0.87083333 0.875 0.87916667 0.88333333 0.8875 0.89166667 0.89583333 0.9 0.90416667 0.90833333 0.9125 0.91666667 0.92083333 0.925 0.92916667 0.93333333 0.9375 0.94166667 0.94583333 0.95 0.95416667 0.95833333 0.9625 0.96666667 0.97083333 0.975 0.97916667 0.98333333 0.9875 0.99166667 0.99583333 1 1 1 1 1 1
  arc A49 (2.755, -18.3773) -> (3.7249, -18.2754) centre (0, 12.5) ccw
  spline S41 degree 5 poles (3.7249, -18.2754) (3.7256, -18.2728) (3.7268, -18.2675) (3.7287, -18.2596) (3.7312, -18.2491) (3.7343, -18.236) (3.7374, -18.223) (3.7405, -18.2099) (3.7435, -18.1969) (3.7466, -18.1839) (3.7496, -18.171) (3.7525, -18.158) (3.7555, -18.1451) (3.7584, -18.1323) (3.7613, -18.1194) (3.7642, -18.1066) (3.767, -18.0938) (3.7699, -18.081) (3.7727, -18.0683) (3.7755, -18.0556) (3.7782, -18.0429) (3.781, -18.0302) (3.7837, -18.0176) (3.7864, -18.005) (3.7891, -17.9924) (3.7917, -17.9799) (3.7943, -17.9674) (3.797, -17.9549) (3.7995, -17.9424) (3.8021, -17.93) (3.8046, -17.9176) (3.8071, -17.9053) (3.8096, -17.8929) (3.8121, -17.8806) (3.8145, -17.8683) (3.817, -17.8561) (3.8194, -17.8439) (3.8217, -17.8317) (3.8241, -17.8195) (3.8264, -17.8074) (3.8288, -17.7953) (3.831, -17.7832) (3.8333, -17.7712) (3.8356, -17.7592) (3.8378, -17.7472) (3.84, -17.7353) (3.8422, -17.7233) (3.8443, -17.7115) (3.8464, -17.6996) (3.8486, -17.6878) (3.8507, -17.676) (3.8527, -17.6643) (3.8548, -17.6525) (3.8568, -17.6409) (3.8588, -17.6292) (3.8608, -17.6176) (3.8628, -17.606) (3.8647, -17.5944) (3.8666, -17.5829) (3.8685, -17.5714) (3.8704, -17.56) (3.8722, -17.5486) (3.8741, -17.5372) (3.8759, -17.5258) (3.8777, -17.5145) (3.8795, -17.5032) (3.8812, -17.492) (3.8829, -17.4807) (3.8846, -17.4696) (3.8863, -17.4584) (3.888, -17.4473) (3.8896, -17.4362) (3.8913, -17.4252) (3.8929, -17.4142) (3.8945, -17.4032) (3.896, -17.3923) (3.8976, -17.3814) (3.8991, -17.3705) (3.9006, -17.3597) (3.9021, -17.3489) (3.9035, -17.3382) (3.905, -17.3274) (3.9064, -17.3168) (3.9078, -17.3061) (3.9092, -17.2955) (3.9106, -17.285) (3.9119, -17.2744) (3.9132, -17.264) (3.9145, -17.2535) (3.9158, -17.2431) (3.9171, -17.2327) (3.9183, -17.2224) (3.9196, -17.2121) (3.9208, -17.2018) (3.922, -17.1916) (3.9231, -17.1814) (3.9243, -17.1713) (3.9254, -17.1612) (3.9265, -17.1512) (3.9276, -17.1411) (3.9287, -17.1312) (3.9297, -17.1212) (3.9308, -17.1113) (3.9318, -17.1015) (3.9328, -17.0917) (3.9338, -17.0819) (3.9348, -17.0722) (3.9357, -17.0625) (3.9366, -17.0529) (3.9375, -17.0433) (3.9384, -17.0337) (3.9393, -17.0242) (3.9402, -17.0147) (3.941, -17.0053) (3.9418, -16.9959) (3.9426, -16.9866) (3.9434, -16.9773) (3.9442, -16.968) (3.9449, -16.9588) (3.9457, -16.9497) (3.9464, -16.9406) (3.9471, -16.9315) (3.9478, -16.9225) (3.9484, -16.9135) (3.9491, -16.9045) (3.9497, -16.8957) (3.9503, -16.8868) (3.9509, -16.878) (3.9515, -16.8693) (3.9521, -16.8606) (3.9526, -16.8519) (3.9532, -16.8433) (3.9537, -16.8348) (3.9542, -16.8263) (3.9547, -16.8178) (3.9552, -16.8094) (3.9556, -16.801) (3.9561, -16.7927) (3.9565, -16.7845) (3.9569, -16.7763) (3.9573, -16.7681) (3.9577, -16.76) (3.9581, -16.7519) (3.9584, -16.7439) (3.9588, -16.736) (3.9591, -16.7281) (3.9594, -16.7202) (3.9597, -16.7124) (3.96, -16.7047) (3.9603, -16.697) (3.9605, -16.6893) (3.9607, -16.6817) (3.961, -16.6742) (3.9612, -16.6667) (3.9614, -16.6593) (3.9616, -16.6519) (3.9618, -16.6446) (3.9619, -16.6374) (3.9621, -16.6302) (3.9622, -16.623) (3.9623, -16.6159) (3.9625, -16.6089) (3.9626, -16.6019) (3.9626, -16.595) (3.9627, -16.5882) (3.9628, -16.5814) (3.9628, -16.5746) (3.9629, -16.568) (3.9629, -16.5613) (3.9629, -16.5548) (3.963, -16.5483) (3.963, -16.5418) (3.9629, -16.5355) (3.9629, -16.5291) (3.9629, -16.5229) (3.9629, -16.5167) (3.9628, -16.5106) (3.9627, -16.5045) (3.9627, -16.4985) (3.9626, -16.4926) (3.9625, -16.4867) (3.9624, -16.4809) (3.9623, -16.4752) (3.9622, -16.4695) (3.9621, -16.4639) (3.962, -16.4584) (3.9618, -16.4529) (3.9617, -16.4475) (3.9615, -16.4422) (3.9614, -16.4369) (3.9612, -16.4317) (3.961, -16.4266) (3.9609, -16.4215) (3.9607, -16.4166) (3.9605, -16.4117) (3.9603, -16.4068) (3.9601, -16.4021) (3.9599, -16.3974) (3.9597, -16.3928) (3.9595, -16.3882) (3.9593, -16.3838) (3.959, -16.3794) (3.9588, -16.3751) (3.9586, -16.3709) (3.9584, -16.3667) (3.9581, -16.3626) (3.9579, -16.3586) (3.9577, -16.3547) (3.9574, -16.3509) (3.9572, -16.3472) (3.9569, -16.3435) (3.9567, -16.3399) (3.9564, -16.3364) (3.9562, -16.333) (3.9559, -16.3297) (3.9557, -16.3264) (3.9555, -16.3233) (3.9552, -16.3202) (3.955, -16.3172) (3.9547, -16.3144) (3.9545, -16.3116) (3.9543, -16.3089) (3.954, -16.3063) (3.9538, -16.3037) (3.9536, -16.3013) (3.9534, -16.299) (3.9531, -16.2968) (3.9529, -16.2946) (3.9527, -16.2926) (3.9525, -16.2907) (3.9523, -16.2889) (3.9522, -16.2871) (3.952, -16.2855) (3.9518, -16.284) (3.9517, -16.2826) (3.9515, -16.2813) (3.9514, -16.2801) (3.9512, -16.279) (3.9511, -16.278) (3.951, -16.2772) (3.9509, -16.2764) (3.9509, -16.2759) (3.9508, -16.2756) (3.9508, -16.2754) (3.9508, -16.2753) knots -1 -1 -1 -1 -1 -1 -0.99583333 -0.99166667 -0.9875 -0.98333333 -0.97916667 -0.975 -0.97083333 -0.96666667 -0.9625 -0.95833333 -0.95416667 -0.95 -0.94583333 -0.94166667 -0.9375 -0.93333333 -0.92916667 -0.925 -0.92083333 -0.91666667 -0.9125 -0.90833333 -0.90416667 -0.9 -0.89583333 -0.89166667 -0.8875 -0.88333333 -0.87916667 -0.875 -0.87083333 -0.86666667 -0.8625 -0.85833333 -0.85416667 -0.85 -0.84583333 -0.84166667 -0.8375 -0.83333333 -0.82916667 -0.825 -0.82083333 -0.81666667 -0.8125 -0.80833333 -0.80416667 -0.8 -0.79583333 -0.79166667 -0.7875 -0.78333333 -0.77916667 -0.775 -0.77083333 -0.76666667 -0.7625 -0.75833333 -0.75416667 -0.75 -0.74583333 -0.74166667 -0.7375 -0.73333333 -0.72916667 -0.725 -0.72083333 -0.71666667 -0.7125 -0.70833333 -0.70416667 -0.7 -0.69583333 -0.69166667 -0.6875 -0.68333333 -0.67916667 -0.675 -0.67083333 -0.66666667 -0.6625 -0.65833333 -0.65416667 -0.65 -0.64583333 -0.64166667 -0.6375 -0.63333333 -0.62916667 -0.625 -0.62083333 -0.61666667 -0.6125 -0.60833333 -0.60416667 -0.6 -0.59583333 -0.59166667 -0.5875 -0.58333333 -0.57916667 -0.575 -0.57083333 -0.56666667 -0.5625 -0.55833333 -0.55416667 -0.55 -0.54583333 -0.54166667 -0.5375 -0.53333333 -0.52916667 -0.525 -0.52083333 -0.51666667 -0.5125 -0.50833333 -0.50416667 -0.5 -0.49583333 -0.49166667 -0.4875 -0.48333333 -0.47916667 -0.475 -0.47083333 -0.46666667 -0.4625 -0.45833333 -0.45416667 -0.45 -0.44583333 -0.44166667 -0.4375 -0.43333333 -0.42916667 -0.425 -0.42083333 -0.41666667 -0.4125 -0.40833333 -0.40416667 -0.4 -0.39583333 -0.39166667 -0.3875 -0.38333333 -0.37916667 -0.375 -0.37083333 -0.36666667 -0.3625 -0.35833333 -0.35416667 -0.35 -0.34583333 -0.34166667 -0.3375 -0.33333333 -0.32916667 -0.325 -0.32083333 -0.31666667 -0.3125 -0.30833333 -0.30416667 -0.3 -0.29583333 -0.29166667 -0.2875 -0.28333333 -0.27916667 -0.275 -0.27083333 -0.26666667 -0.2625 -0.25833333 -0.25416667 -0.25 -0.24583333 -0.24166667 -0.2375 -0.23333333 -0.22916667 -0.225 -0.22083333 -0.21666667 -0.2125 -0.20833333 -0.20416667 -0.2 -0.19583333 -0.19166667 -0.1875 -0.18333333 -0.17916667 -0.175 -0.17083333 -0.16666667 -0.1625 -0.15833333 -0.15416667 -0.15 -0.14583333 -0.14166667 -0.1375 -0.13333333 -0.12916667 -0.125 -0.12083333 -0.11666667 -0.1125 -0.10833333 -0.10416667 -0.1 -0.09583333 -0.09166667 -0.0875 -0.08333333 -0.07916667 -0.075 -0.07083333 -0.06666667 -0.0625 -0.05833333 -0.05416667 -0.05 -0.04583333 -0.04166667 -0.0375 -0.03333333 -0.02916667 -0.025 -0.02083333 -0.01666667 -0.0125 -0.00833333 -0.00416667 0 0 0 0 0 0
  line L83 (3.9508, -16.2753) -> (3.9507, -16.2745)
  line L84 (3.9507, -16.2745) -> (3.9106, -15.9828)
  arc A50 (3.9106, -15.9828) -> (5.0824, -15.7972) centre (0, 12.5) ccw
  line L85 (5.0824, -15.7972) -> (5.1345, -16.087)
  line L86 (5.1345, -16.087) -> (5.1346, -16.0878)